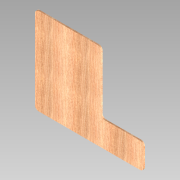
# Autodesk Inventor part: 4102_Mounting Plate_V1
Saved by Autodesk Inventor 2020 (Build 240168000, 168)
## iProperties
Created: 2020-09-10
Part Number: 4102_Mounting Plate_V1
Material: Wood (Birch)
Document SubType Name: Modeling
Designer: Eli Mattingly
Density: 0.55 g/cm^3
Appearance: Birch - Natural Polished
Author: Eli Mattingly
Autodesk Inventor part; units mm, degrees
ref_plane "YZ Plane" through (0, 0, 0) normal (1, 0, 0) x (0, 1, 0)
ref_plane "XZ Plane" through (0, 0, 0) normal (0, 1, 0) x (-1, 0, 0)
ref_plane "XY Plane" through (0, 0, 0) normal (0, 0, 1) x (1, 0, 0)
sketch "Sketch1" plane through (0, 0, 0) normal (0, 0, 1) x (1, 0, 0)
  line L0 (-375, 300) -> (375, 300)
  line L1 (375, 300) -> (375, -300)
  line L2 (375, -300) -> (-375, -300)
  line L3 (-375, -300) -> (-375, 300)
  line L4 (-375, 300) -> (375, -300) construction
  line L5 (375, 300) -> (-375, -300) construction
  line L6 (375, 300) -> (82.2, 300)
  line L7 (82.2, 300) -> (82.2, -125)
  line L8 (82.2, -125) -> (375, -125)
  line L9 (375, -125) -> (375, 300)
  point P0 (0, 0)
  point P1 (375, -125)
  point P2 (82.2, 300)
  dimension "d0" = 750
  dimension "d1" = 600
  dimension "d2" = 457.2
  dimension "d3" = 175
  constraints: 20 end point, 4 parallel, 2 horizontal, 2 midpoint, 2 perpendicular
  measures "d0" distance of L1.end L2.end
  measures "d1" distance of L0.end L1.end
  measures "d2" distance between parallel lines of L3 L7
  measures "d3" distance between parallel lines of L2 L8
extrude "Extrusion1" add sketch "Sketch1" along normal blind 10 contours L0 L7 L8 L1 L2 L3
fillet "Fillet1" radius 25 6 edges at (82.2, -125, 5) (375, -125, 5) (375, -300, 5) (-375, -300, 5) (-375, 300, 5) (82.2, 300, 5)
body "Solid1"
